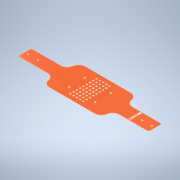
# Autodesk Inventor part: Flex
Saved by Autodesk Inventor 2022 (Build 260153000, 153)
## iProperties
Created: 2021-07-16
Part Number: Flex
Material: Phenolic Resin
Document SubType Name: Modeling
Designer: Caleb
Density: 1.38 g/cm^3
Appearance: Smooth - Light Orange
Author: Caleb
Autodesk Inventor part; units mm, degrees
ref_plane "YZ Plane" through (0, 0, 0) normal (1, 0, 0) x (0, 1, 0)
ref_plane "XZ Plane" through (0, 0, 0) normal (0, 1, 0) x (-1, 0, 0)
ref_plane "XY Plane" through (0, 0, 0) normal (0, 0, 1) x (1, 0, 0)
sketch "Sketch1" plane through (0, 0, 0) normal (0, 1, 0) x (-1, 0, 0)
  line L0 (-22.15, 17.5) -> (22.15, 17.5)
  line L1 (28.5, 11.15) -> (28.5, 12.7)
  line L2 (22.15, -17.5) -> (-22.15, -17.5)
  line L3 (-28.5, 12.7) -> (-28.5, 11.15)
  line L4 (-28.5, 17.5) -> (28.5, -17.5) construction
  line L5 (28.5, 17.5) -> (-28.5, -17.5) construction
  line L6 (34.85, -6.35) -> (61.9137, -6.35)
  line L7 (63.5012, -4.7625) -> (63.5012, 4.7625)
  line L8 (61.9137, 6.35) -> (34.85, 6.35)
  line L9 (-34.85, -6.35) -> (-61.9137, -6.35)
  line L10 (-63.5012, -4.7625) -> (-63.5012, 4.7625)
  line L11 (-61.9137, 6.35) -> (-34.85, 6.35)
  arc A0 (28.5, 11.15) -> (22.15, 17.5) centre (22.15, 11.15) ccw
  arc A1 (22.15, -17.5) -> (28.5, -11.15) centre (22.15, -11.15) ccw
  arc A2 (-28.5, -11.15) -> (-22.15, -17.5) centre (-22.15, -11.15) ccw
  arc A3 (-22.15, 17.5) -> (-28.5, 11.15) centre (-22.15, 11.15) ccw
  arc A4 (-34.85, 6.35) -> (-28.5, 12.7) centre (-34.85, 12.7) ccw
  arc A5 (28.5, 12.7) -> (34.85, 6.35) centre (34.85, 12.7) ccw
  line L12 (-28.5, -12.7) -> (-28.5, -11.15)
  line L13 (28.5, -12.7) -> (28.5, -11.15)
  arc A6 (34.85, -6.35) -> (28.5, -12.7) centre (34.85, -12.7) ccw
  arc A7 (-28.5, -12.7) -> (-34.85, -6.35) centre (-34.85, -12.7) ccw
  arc A8 (61.9137, -6.35) -> (63.5012, -4.7625) centre (61.9137, -4.7625) ccw
  arc A9 (63.5012, 4.7625) -> (61.9137, 6.35) centre (61.9137, 4.7625) ccw
  arc A10 (-63.5012, -4.7625) -> (-61.9137, -6.35) centre (-61.9137, -4.7625) ccw
  arc A11 (-61.9137, 6.35) -> (-63.5012, 4.7625) centre (-61.9137, 4.7625) ccw
  point P0 (0, 0)
  point P1 (28.5, -6.35)
  point P2 (63.5012, 6.35)
  point P3 (63.5012, -6.35)
  point P4 (-28.5, -6.35)
  point P5 (-63.5012, 6.35)
  point P6 (-63.5012, -6.35)
  dimension "d0" = 57
  dimension "d1" = 35
  dimension "d2" = 35.0012
  dimension "d3" = 12.7
  dimension "d4" = 6.35
  dimension "d5" = 6.35
  dimension "d6" = 6.35
  dimension "d7" = 6.35
  dimension "d8" = 6.35
  dimension "d9" = 6.35
  dimension "d10" = 6.35
  dimension "d13" = 1.5875
  constraints: 28 end point, 26 point on line, 25 point on circle, 24 tangent, 12 centre point, 5 equal radius, 4 parallel, 3 horizontal, 3 perpendicular, 2 midpoint, 2 vertical, 1 collinear
  measures "d0" distance of L4.end L5.end
  measures "d1" distance of L5.end L4.start
  measures "d2" distance of point (-28.5, -6.35) point (-63.501, -6.35)
  measures "d3" distance of point (-63.501, -6.35) point (-63.501, 6.35)
  measures "d4" distance from line of L11 point (0, 0)
  measures "d5" radius of A0
  measures "d6" radius of A1
  measures "d7" radius of A2
  measures "d8" radius of A3
  measures "d9" radius of A4
  measures "d10" radius of A6
  measures "d13" radius of A8
extrude "Extrusion1" add sketch "Sketch1" along normal blind 0.12
sketch "Sketch2" plane through (0, 0.12, 0) normal (0, 1, 0) x (1, 0, 0)
  line L0 (-63.5012, 4.7625) -> (-63.5012, -4.7625) projected
  line L1 (63.5012, -4.7625) -> (63.5012, 4.7625) projected
  point P0 (0, 0)
  point P1 (-50.8012, 0)
  point P2 (50.8012, 0)
  point P3 (-60.3262, 0)
  point P4 (60.3262, 0)
  point P5 (-12.7012, 7.62)
  point P6 (-12.7012, -7.62)
  point P7 (12.7012, 7.62)
  point P8 (12.7012, -7.62)
  dimension "d14" = 12.7
  dimension "d15" = 12.7
  dimension "d23" = 3.175
  dimension "d24" = 3.175
  dimension "d46" = 50.8
  dimension "d47" = 50.8
  dimension "d48" = 7.62
  dimension "d49" = 7.62
  constraints: 2 horizontal alignment, 2 vertical alignment
  measures "d14" distance from line of L0 point (-50.801, 0)
  measures "d15" distance from line of L1 point (50.801, 0)
  measures "d23" distance from line of L0 point (-60.326, 0)
  measures "d24" distance from line of L1 point (60.326, 0)
  measures "d46" distance from line of point (-12.701, 7.62) L0
  measures "d47" distance from line of point (12.701, 7.62) L1
  measures "d48" vertical distance of point (-12.701, 7.62) point (0, 0)
  measures "d49" vertical distance of point (-12.701, -7.62) point (0, 0)
hole "Hole1" at (-50.8012, 0.12, 0) at (50.8012, 0.12, 0) at (-60.3262, 0.12, 0) at (60.3262, 0.12, 0) at (-12.7012, 0.12, -7.62) at (-12.7012, 0.12, 7.62) at (12.7012, 0.12, -7.62) at (12.7012, 0.12, 7.62) direction (0, -1, 0) diameter 1.6256 end through all clearance for "Flat Head Machine Screw (82)" size "#0" standard "Ansi Unified Screw Threads"
sketch "Sketch3" plane through (0, 0.12, 0) normal (0, 1, 0) x (1, 0, 0)
  line L0 (-7.6554, 0) -> (0, 0)
  line L1 (0, 0) -> (0, -7.3938)
  point P0 (-6.35, -12.7)
  point P1 (-6.35, -9.525)
  point P2 (-6.35, -6.35)
  point P3 (-6.35, -3.175)
  point P4 (-6.35, 0)
  point P5 (-6.35, 3.175)
  point P6 (-6.35, 6.35)
  point P7 (-6.35, 9.525)
  point P8 (-6.35, 12.7)
  point P9 (-3.175, -12.7)
  point P10 (-3.175, -9.525)
  point P11 (-3.175, -6.35)
  point P12 (-3.175, -3.175)
  point P13 (-3.175, 0)
  point P14 (-3.175, 3.175)
  point P15 (-3.175, 6.35)
  point P16 (-3.175, 9.525)
  point P17 (-3.175, 12.7)
  point P18 (0, -12.7)
  point P19 (0, -9.525)
  point P20 (0, -6.35)
  point P21 (0, -3.175)
  point P22 (0, 3.175)
  point P23 (0, 6.35)
  point P24 (0, 9.525)
  point P25 (0, 12.7)
  point P26 (3.175, -12.7)
  point P27 (3.175, -9.525)
  point P28 (3.175, -6.35)
  point P29 (3.175, -3.175)
  point P30 (3.175, 0)
  point P31 (3.175, 3.175)
  point P32 (3.175, 6.35)
  point P33 (3.175, 9.525)
  point P34 (3.175, 12.7)
  point P35 (6.35, -12.7)
  point P36 (6.35, -9.525)
  point P37 (6.35, -6.35)
  point P38 (6.35, -3.175)
  point P39 (6.35, 0)
  point P40 (6.35, 3.175)
  point P41 (6.35, 6.35)
  point P42 (6.35, 9.525)
  point P43 (6.35, 12.7)
  dimension "d25" = 12.7
  dimension "d26" = 6.35
  dimension "d29" = 3.175
  dimension "d32" = 3.175
  constraints: 4 end point, 2 horizontal, 1 perpendicular, 1 vertical, 44 other
  measures "d25" vertical distance of L0.end point (-6.35, -12.7)
  measures "d26" horizontal distance of point (-6.35, -12.7) L0.end
  measures "d29" distance of point (-6.35, -12.7) point (-6.35, -9.525)
  measures "d32" distance of point (-6.35, -12.7) point (-3.175, -12.7)
hole "Hole2" at (-6.35, 0.12, 12.7) at (-6.35, 0.12, 9.525) at (-6.35, 0.12, 6.35) at (-6.35, 0.12, 3.175) at (-6.35, 0.12, 0) at (-6.35, 0.12, -3.175) at (-6.35, 0.12, -6.35) at (-6.35, 0.12, -9.525) at (-6.35, 0.12, -12.7) at (-3.175, 0.12, 12.7) at (-3.175, 0.12, 9.525) at (-3.175, 0.12, 6.35) at (-3.175, 0.12, 3.175) at (-3.175, 0.12, 0) at (-3.175, 0.12, -3.175) at (-3.175, 0.12, -6.35) at (-3.175, 0.12, -9.525) at (-3.175, 0.12, -12.7) at (0, 0.12, 12.7) at (0, 0.12, 9.525) at (0, 0.12, 6.35) at (0, 0.12, 3.175) at (0, 0.12, 0) at (0, 0.12, -3.175) at (0, 0.12, -6.35) at (0, 0.12, -9.525) at (0, 0.12, -12.7) at (3.175, 0.12, 12.7) at (3.175, 0.12, 9.525) at (3.175, 0.12, 6.35) at (3.175, 0.12, 3.175) at (3.175, 0.12, 0) at (3.175, 0.12, -3.175) at (3.175, 0.12, -6.35) at (3.175, 0.12, -9.525) at (3.175, 0.12, -12.7) at (6.35, 0.12, 12.7) at (6.35, 0.12, 9.525) at (6.35, 0.12, 6.35) at (6.35, 0.12, 3.175) at (6.35, 0.12, 0) at (6.35, 0.12, -3.175) at (6.35, 0.12, -6.35) at (6.35, 0.12, -9.525) at (6.35, 0.12, -12.7) direction (0, -1, 0) diameter 1.5875 end through all
sketch "Sketch4" plane through (0, 0.12, 0) normal (0, 1, 0) x (1, 0, 0)
  line L0 (44.9128, -5.6293) -> (42.91, -5.6293)
  line L1 (42.91, -5.6293) -> (42.91, 5.6293)
  line L2 (42.91, 5.6293) -> (44.9128, 5.6293)
  line L3 (44.9128, 5.6293) -> (44.9128, -5.6293)
  line L4 (44.9128, -5.6293) -> (42.91, 5.6293) construction
  line L5 (42.91, -5.6293) -> (44.9128, 5.6293) construction
  point P0 (0, 0)
  point P1 (43.9114, 0)
  constraints: 12 end point, 2 midpoint, 2 parallel, 1 horizontal, 1 perpendicular
extrude "Extrusion2" add sketch "Sketch4" along normal blind 0.05
sketch "Sketch5" plane through (0, 0.17, 0) normal (0, 1, 0) x (1, 0, 0)
  line L0 (43.0643, -5.3096) -> (43.0643, 12.5684) construction
  line L1 (43.0643, 12.5684) -> (46.2383, 12.5684) construction
  line L2 (46.2383, 12.5684) -> (46.2383, -5.3096) construction
  line L3 (46.2383, -5.3096) -> (43.0643, -5.3096) construction
  spline S0 degree 2 poles (44.6464, -4.7304) (44.6464, -4.8958) (44.5772, -5.128) (44.5278, -5.2305) knots 0 0 0 1 2 2 2
  line L4 (44.5278, -5.2305) -> (44.2734, -5.2305)
  line L5 (44.2734, -5.2305) -> (44.2734, -5.2157)
  spline S1 degree 2 poles (44.2734, -5.2157) (44.3673, -5.1157) (44.471, -4.8625) (44.471, -4.7452) knots 0 0 0 1 2 2 2
  spline S2 degree 2 poles (44.471, -4.7452) (44.471, -4.5772) (44.3314, -4.4055) (44.2166, -4.4055) knots 0 0 0 1 2 2 2
  spline S3 degree 2 poles (44.2166, -4.4055) (44.1252, -4.4055) (44.0116, -4.4957) (43.9832, -4.5933) knots 0 0 0 1 2 2 2
  spline S4 degree 2 poles (43.9832, -4.5933) (43.9634, -4.6637) (43.9362, -4.781) (43.914, -4.8687) knots 0 0 0 1 2 2 2
  spline S5 degree 2 poles (43.914, -4.8687) (43.893, -4.9477) (43.83, -5.0725) (43.7794, -5.1206) knots 0 0 0 1 2 2 2
  spline S6 degree 2 poles (43.7794, -5.1206) (43.7288, -5.1675) (43.5929, -5.2194) (43.504, -5.2194) knots 0 0 0 1 2 2 2
  spline S7 degree 2 poles (43.504, -5.2194) (43.3187, -5.2194) (43.068, -4.9304) (43.068, -4.7069) knots 0 0 0 1 2 2 2
  spline S8 degree 2 poles (43.068, -4.7069) (43.068, -4.5784) (43.1187, -4.3512) (43.1668, -4.2536) knots 0 0 0 1 2 2 2
  line L6 (43.1668, -4.2536) -> (43.4089, -4.2536)
  line L7 (43.4089, -4.2536) -> (43.4089, -4.2685)
  spline S9 degree 2 poles (43.4089, -4.2685) (43.3422, -4.3413) (43.2434, -4.5686) (43.2434, -4.6933) knots 0 0 0 1 2 2 2
  spline S10 degree 2 poles (43.2434, -4.6933) (43.2434, -4.8341) (43.3755, -5.0082) (43.483, -5.0082) knots 0 0 0 1 2 2 2
  spline S11 degree 2 poles (43.483, -5.0082) (43.5793, -5.0082) (43.6942, -4.9057) (43.7201, -4.8094) knots 0 0 0 1 2 2 2
  spline S12 degree 2 poles (43.7201, -4.8094) (43.7374, -4.7452) (43.7819, -4.5587) (43.8004, -4.4969) knots 0 0 0 1 2 2 2
  spline S13 degree 2 poles (43.8004, -4.4969) (43.8486, -4.3401) (44.0424, -4.1944) (44.1845, -4.1944) knots 0 0 0 1 2 2 2
  spline S14 degree 2 poles (44.1845, -4.1944) (44.2746, -4.1944) (44.4475, -4.2672) (44.508, -4.3327) knots 0 0 0 1 2 2 2
  spline S15 degree 2 poles (44.508, -4.3327) (44.5747, -4.4055) (44.6464, -4.5908) (44.6464, -4.7304) knots 0 0 0 1 2 2 2
  line L8 (44.6192, -2.8976) -> (44.6192, -3.1248)
  line L9 (44.6192, -3.1248) -> (43.3051, -3.7992)
  line L10 (43.3051, -3.7992) -> (44.6192, -3.7992)
  line L11 (44.6192, -3.7992) -> (44.6192, -3.9881)
  line L12 (44.6192, -3.9881) -> (43.0952, -3.9881)
  line L13 (43.0952, -3.9881) -> (43.0952, -3.7004)
  line L14 (43.0952, -3.7004) -> (44.3018, -3.0866)
  line L15 (44.3018, -3.0866) -> (43.0952, -3.0866)
  line L16 (43.0952, -3.0866) -> (43.0952, -2.8976)
  line L17 (43.0952, -2.8976) -> (44.6192, -2.8976)
  spline S16 degree 2 poles (43.8572, -1.029) (44.2672, -1.029) (44.6513, -1.2674) (44.6513, -1.5156) knots 0 0 0 1 2 2 2
  spline S17 degree 2 poles (44.6513, -1.5156) (44.6513, -1.7676) (44.2598, -2.0035) (43.8584, -2.0035) knots 0 0 0 1 2 2 2
  spline S18 degree 2 poles (43.8584, -2.0035) (43.4459, -2.0035) (43.0643, -1.7651) (43.0643, -1.5156) knots 0 0 0 1 2 2 2
  spline S19 degree 2 poles (43.0643, -1.5156) (43.0643, -1.2649) (43.4595, -1.029) (43.8572, -1.029) knots 0 0 0 1 2 2 2
  spline S20 degree 2 poles (44.3216, -1.2909) (44.2462, -1.2612) (44.014, -1.2365) (43.8572, -1.2365) knots 0 0 0 1 2 2 2
  spline S21 degree 2 poles (43.8572, -1.2365) (43.7003, -1.2365) (43.4694, -1.2612) (43.3916, -1.2921) knots 0 0 0 1 2 2 2
  spline S22 degree 2 poles (43.3916, -1.2921) (43.3138, -1.323) (43.2335, -1.4304) (43.2335, -1.5156) knots 0 0 0 1 2 2 2
  spline S23 degree 2 poles (43.2335, -1.5156) (43.2335, -1.6008) (43.3138, -1.7108) (43.3941, -1.7429) knots 0 0 0 1 2 2 2
  spline S24 degree 2 poles (43.3941, -1.7429) (43.4719, -1.7737) (43.709, -1.796) (43.8584, -1.796) knots 0 0 0 1 2 2 2
  spline S25 degree 2 poles (43.8584, -1.796) (44.019, -1.796) (44.2339, -1.7762) (44.3179, -1.7441) knots 0 0 0 1 2 2 2
  spline S26 degree 2 poles (44.3179, -1.7441) (44.3969, -1.7145) (44.4821, -1.6045) (44.4821, -1.5156) knots 0 0 0 1 2 2 2
  spline S27 degree 2 poles (44.4821, -1.5156) (44.4821, -1.4316) (44.4018, -1.3217) (44.3216, -1.2909) knots 0 0 0 1 2 2 2
  spline S28 degree 2 poles (43.8572, 0.1146) (44.2672, 0.1146) (44.6513, -0.1238) (44.6513, -0.372) knots 0 0 0 1 2 2 2
  spline S29 degree 2 poles (44.6513, -0.372) (44.6513, -0.624) (44.2598, -0.8598) (43.8584, -0.8598) knots 0 0 0 1 2 2 2
  spline S30 degree 2 poles (43.8584, -0.8598) (43.4459, -0.8598) (43.0643, -0.6215) (43.0643, -0.372) knots 0 0 0 1 2 2 2
  spline S31 degree 2 poles (43.0643, -0.372) (43.0643, -0.1213) (43.4595, 0.1146) (43.8572, 0.1146) knots 0 0 0 1 2 2 2
  spline S32 degree 2 poles (44.3216, -0.1472) (44.2462, -0.1176) (44.014, -0.0929) (43.8572, -0.0929) knots 0 0 0 1 2 2 2
  spline S33 degree 2 poles (43.8572, -0.0929) (43.7003, -0.0929) (43.4694, -0.1176) (43.3916, -0.1485) knots 0 0 0 1 2 2 2
  spline S34 degree 2 poles (43.3916, -0.1485) (43.3138, -0.1793) (43.2335, -0.2868) (43.2335, -0.372) knots 0 0 0 1 2 2 2
  spline S35 degree 2 poles (43.2335, -0.372) (43.2335, -0.4572) (43.3138, -0.5671) (43.3941, -0.5993) knots 0 0 0 1 2 2 2
  spline S36 degree 2 poles (43.3941, -0.5993) (43.4719, -0.6301) (43.709, -0.6524) (43.8584, -0.6524) knots 0 0 0 1 2 2 2
  spline S37 degree 2 poles (43.8584, -0.6524) (44.019, -0.6524) (44.2339, -0.6326) (44.3179, -0.6005) knots 0 0 0 1 2 2 2
  spline S38 degree 2 poles (44.3179, -0.6005) (44.3969, -0.5708) (44.4821, -0.4609) (44.4821, -0.372) knots 0 0 0 1 2 2 2
  spline S39 degree 2 poles (44.4821, -0.372) (44.4821, -0.288) (44.4018, -0.1781) (44.3216, -0.1472) knots 0 0 0 1 2 2 2
  spline S40 degree 2 poles (43.8572, 1.2582) (44.2672, 1.2582) (44.6513, 1.0198) (44.6513, 0.7716) knots 0 0 0 1 2 2 2
  spline S41 degree 2 poles (44.6513, 0.7716) (44.6513, 0.5197) (44.2598, 0.2838) (43.8584, 0.2838) knots 0 0 0 1 2 2 2
  spline S42 degree 2 poles (43.8584, 0.2838) (43.4459, 0.2838) (43.0643, 0.5221) (43.0643, 0.7716) knots 0 0 0 1 2 2 2
  spline S43 degree 2 poles (43.0643, 0.7716) (43.0643, 1.0223) (43.4595, 1.2582) (43.8572, 1.2582) knots 0 0 0 1 2 2 2
  spline S44 degree 2 poles (44.3216, 0.9964) (44.2462, 1.026) (44.014, 1.0507) (43.8572, 1.0507) knots 0 0 0 1 2 2 2
  spline S45 degree 2 poles (43.8572, 1.0507) (43.7003, 1.0507) (43.4694, 1.026) (43.3916, 0.9951) knots 0 0 0 1 2 2 2
  spline S46 degree 2 poles (43.3916, 0.9951) (43.3138, 0.9643) (43.2335, 0.8568) (43.2335, 0.7716) knots 0 0 0 1 2 2 2
  spline S47 degree 2 poles (43.2335, 0.7716) (43.2335, 0.6864) (43.3138, 0.5765) (43.3941, 0.5444) knots 0 0 0 1 2 2 2
  spline S48 degree 2 poles (43.3941, 0.5444) (43.4719, 0.5135) (43.709, 0.4913) (43.8584, 0.4913) knots 0 0 0 1 2 2 2
  spline S49 degree 2 poles (43.8584, 0.4913) (44.019, 0.4913) (44.2339, 0.511) (44.3179, 0.5431) knots 0 0 0 1 2 2 2
  spline S50 degree 2 poles (44.3179, 0.5431) (44.3969, 0.5728) (44.4821, 0.6827) (44.4821, 0.7716) knots 0 0 0 1 2 2 2
  spline S51 degree 2 poles (44.4821, 0.7716) (44.4821, 0.8556) (44.4018, 0.9655) (44.3216, 0.9964) knots 0 0 0 1 2 2 2
  spline S52 degree 2 poles (43.8572, 2.4018) (44.2672, 2.4018) (44.6513, 2.1635) (44.6513, 1.9152) knots 0 0 0 1 2 2 2
  spline S53 degree 2 poles (44.6513, 1.9152) (44.6513, 1.6633) (44.2598, 1.4274) (43.8584, 1.4274) knots 0 0 0 1 2 2 2
  spline S54 degree 2 poles (43.8584, 1.4274) (43.4459, 1.4274) (43.0643, 1.6658) (43.0643, 1.9152) knots 0 0 0 1 2 2 2
  spline S55 degree 2 poles (43.0643, 1.9152) (43.0643, 2.1659) (43.4595, 2.4018) (43.8572, 2.4018) knots 0 0 0 1 2 2 2
  spline S56 degree 2 poles (44.3216, 2.14) (44.2462, 2.1696) (44.014, 2.1943) (43.8572, 2.1943) knots 0 0 0 1 2 2 2
  spline S57 degree 2 poles (43.8572, 2.1943) (43.7003, 2.1943) (43.4694, 2.1696) (43.3916, 2.1388) knots 0 0 0 1 2 2 2
  spline S58 degree 2 poles (43.3916, 2.1388) (43.3138, 2.1079) (43.2335, 2.0004) (43.2335, 1.9152) knots 0 0 0 1 2 2 2
  spline S59 degree 2 poles (43.2335, 1.9152) (43.2335, 1.83) (43.3138, 1.7201) (43.3941, 1.688) knots 0 0 0 1 2 2 2
  spline S60 degree 2 poles (43.3941, 1.688) (43.4719, 1.6571) (43.709, 1.6349) (43.8584, 1.6349) knots 0 0 0 1 2 2 2
  spline S61 degree 2 poles (43.8584, 1.6349) (44.019, 1.6349) (44.2339, 1.6546) (44.3179, 1.6867) knots 0 0 0 1 2 2 2
  spline S62 degree 2 poles (44.3179, 1.6867) (44.3969, 1.7164) (44.4821, 1.8263) (44.4821, 1.9152) knots 0 0 0 1 2 2 2
  spline S63 degree 2 poles (44.4821, 1.9152) (44.4821, 1.9992) (44.4018, 2.1091) (44.3216, 2.14) knots 0 0 0 1 2 2 2
  line L18 (44.6192, 3.4602) -> (44.6192, 2.7167)
  line L19 (44.6192, 2.7167) -> (44.4636, 2.7167)
  line L20 (44.4636, 2.7167) -> (44.4636, 2.9934)
  line L21 (44.4636, 2.9934) -> (43.4422, 2.9934)
  line L22 (43.4422, 2.9934) -> (43.4422, 2.7167)
  line L23 (43.4422, 2.7167) -> (43.3027, 2.7167)
  spline S64 degree 2 poles (43.3027, 2.7167) (43.3027, 2.8736) (43.2138, 3.0218) (43.0903, 3.0317) knots 0 0 0 1 2 2 2
  line L24 (43.0903, 3.0317) -> (43.0903, 3.1898)
  line L25 (43.0903, 3.1898) -> (44.4636, 3.1898)
  line L26 (44.4636, 3.1898) -> (44.4636, 3.4602)
  line L27 (44.4636, 3.4602) -> (44.6192, 3.4602)
  point P0 (0, 0)
  constraints: 2 other
emboss "Emboss1" sketch "Sketch5" operation cut depth 0.05 direction (0, -1, 0)
body "Solid1"
